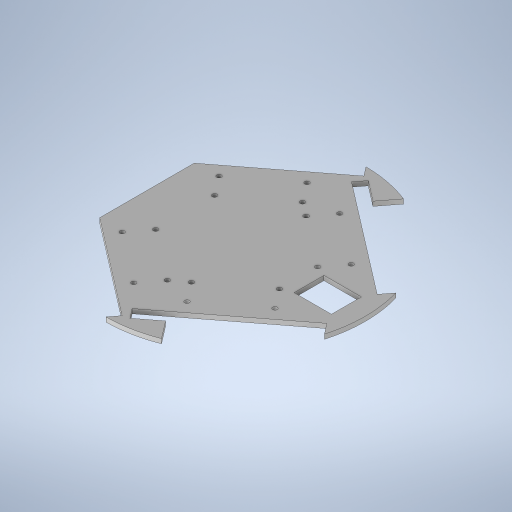
# Autodesk Inventor part: newbasecentral
Saved by Autodesk Inventor 2023.1 (Build 271208000, 208)
## iProperties
Created: 2022-09-07
Part Number: newbasecentral
Material: Genérico
Document SubType Name: Modeling
Designer: Lab. de Manufactura
Density: 1 g/cm^3
Appearance: Valor por defecto
Author: Lab. de Manufactura
Autodesk Inventor part; units mm, degrees
ref_plane "YZ Plane" through (0, 0, 0) normal (1, 0, 0) x (0, 1, 0)
ref_plane "XZ Plane" through (0, 0, 0) normal (0, 1, 0) x (-1, 0, 0)
ref_plane "XY Plane" through (0, 0, 0) normal (0, 0, 1) x (1, 0, 0)
sketch "Boceto1" plane through (0, 0, 0) normal (0, 1, 0) x (-1, 0, 0)
  line L0 (0, 0) -> (0, -87) construction
  line L1 (0, 0) -> (0, 83.8978) construction
  line L2 (0, 0) -> (-87, 0) construction
  line L3 (0, 0) -> (59, 0) construction
  line L4 (-74.5, -10) -> (-49.5, -10)
  line L5 (-49.5, -10) -> (-49.5, 10)
  line L6 (-49.5, 10) -> (-74.5, 10)
  line L7 (-74.5, 10) -> (-74.5, -10)
  line L8 (-74.5, -10) -> (-49.5, 10) construction
  line L9 (-49.5, -10) -> (-74.5, 10) construction
  line L10 (-18, 63.0769) -> (-64.0145, 27.7688)
  line L11 (9, 69.9829) -> (55.0145, 34.6747)
  line L12 (9, 69.9829) -> (20.2282, 84.6157)
  line L13 (-18, 63.0769) -> (-31.752, 80.9988)
  line L14 (-64.0145, 27.7688) -> (-75.6609, 42.9467)
  line L15 (-18, -63.0769) -> (-64.0145, -27.7688)
  line L16 (9, -69.9829) -> (55.0145, -34.6747)
  line L17 (9, -69.9829) -> (20.2282, -84.6157)
  line L18 (-18, -63.0769) -> (-31.752, -80.9988)
  line L19 (-64.0145, -27.7688) -> (-75.6609, -42.9467)
  arc A0 (-75.6609, 42.9467) -> (-75.6609, -42.9467) centre (0, 0) ccw
  arc A1 (20.2282, 84.6157) -> (-31.752, 80.9988) centre (0, 0) ccw
  arc A2 (-31.752, -80.9988) -> (20.2282, -84.6157) centre (0, 0) ccw
  line L20 (59, 37.9189) -> (59, -37.9189)
  line L21 (58.0583, 38.6415) -> (59, 37.9189)
  line L22 (55.0145, 34.6747) -> (58.0583, 38.6415)
  line L23 (58.0583, -38.6415) -> (59, -37.9189)
  line L24 (55.0145, -34.6747) -> (58.0583, -38.6415)
  circle A3 centre (-18.868, 51.0667) radius 1.5
  circle A4 centre (-52.1888, 25.4987) radius 1.5
  line L25 (-41.0072, 45.4229) -> (-35.5284, 38.2827) construction
  line L26 (-18.868, 51.0667) -> (-52.1888, 25.4987) construction
  line L27 (32.0072, 52.3288) -> (22.9685, 40.5493) construction
  circle A5 centre (9.868, 57.9726) radius 1.5
  circle A6 centre (43.1888, 32.4046) radius 1.5
  circle A7 centre (-18.868, -51.0667) radius 1.5
  circle A8 centre (-52.1888, -25.4987) radius 1.5
  circle A9 centre (9.868, -57.9726) radius 1.5
  circle A10 centre (43.1888, -32.4046) radius 1.5
  line L28 (43.1888, 32.4046) -> (9.868, 57.9726) construction
  point P0 (-62, 0)
  point P1 (-74.5, 0)
  point P2 (26.5284, 45.1886)
  dimension "d1" = 25
  dimension "d2" = 20
  dimension "d9" = 52.5
  dimension "d10" = 52.5
  dimension "d11" = 61
  dimension "d12" = 61
  dimension "d13" = 58
  dimension "d17" = 90
  dimension "d18" = 9
  dimension "d19" = 18
  dimension "d20" = 58
  dimension "d21" = 90
  dimension "d22" = 90
  dimension "d23" = 87
  dimension "d24" = 87
  dimension "d26" = 59
  dimension "d27" = 5
  dimension "d28" = 5
  dimension "d29" = 3
  dimension "d30" = 3
  dimension "d31" = 42
  dimension "d32" = 9
  dimension "d37" = 90
  dimension "d38" = 3
  dimension "d39" = 3
  dimension "d40" = 42
  dimension "d41" = 9
  dimension "d54" = 62
  constraints: 58 end point, 11 centre point, 11 symmetric about line, 9 parallel, 8 point on circle, 7 midpoint, 3 horizontal, 3 vertical, 2 perpendicular, 2 point on line, 1 coincident, 4 other
  measures "d1" distance of L5.end L6.end
  measures "d2" distance of L4.end L5.end
  measures "d9" angle of L1 L11
  measures "d10" angle of L1 L10
  measures "d11" distance from line of point (0, 0) L11
  measures "d12" distance from line of point (0, 0) L10
  measures "d13" distance of L11.start L11.end
  measures "d17" angle of L11 L12
  measures "d18" distance from line of L1 L11.start
  measures "d19" distance from line of L1 L10.start
  measures "d20" distance of L10.start L10.end
  measures "d21" angle of L10 L13
  measures "d22" angle of L10 L14
  measures "d23" radius of A0
  measures "d24" radius of A1
  measures "d26" distance between parallel lines of L0 L20
  measures "d27" distance between parallel lines of L11 L21
  measures "d28" distance between parallel lines of L23 L16
  measures "d29" diameter of A3
  measures "d30" diameter of A4
  measures "d31" distance of L26.end L26.start
  measures "d32" distance from line of L10 L26.start
  measures "d37" angle of L11 L27
  measures "d38" diameter of A5
  measures "d39" diameter of A6
  measures "d40" distance of L28.end L28.start
  measures "d41" distance from line of L11 L28.end
  measures "d54" distance of point (0, 0) point (-62, 0)
extrude "Extrusión1" add sketch "Boceto1" along normal blind 3
sketch "Boceto2" plane through (0, 3, 0) normal (0, 1, 0) x (1, 0, 0)
  line L0 (-55.0145, -34.6747) -> (-9, -69.9829) projected
  line L1 (-32.0072, -52.3288) -> (-0.1642, -10.8301) construction
  circle A0 centre (-33.4486, -19.711) radius 1.55
  circle A1 centre (-0.1278, -45.2789) radius 1.55
  line L2 (-33.4486, -19.711) -> (-0.1278, -45.2789) construction
  circle A2 centre (-43.1888, -32.4046) radius 1.5 construction
  line L3 (18, -63.0769) -> (64.0145, -27.7688) projected
  line L4 (41.0072, -45.4229) -> (14.3892, -10.7335) construction
  circle A3 centre (9.1278, -38.373) radius 1.55
  circle A4 centre (42.4486, -12.805) radius 1.55
  line L5 (42.4486, -12.805) -> (9.1278, -38.373) construction
  circle A5 centre (18.868, -51.0667) radius 1.5 construction
  line L6 (-59, 37.9189) -> (-59, -37.9189) construction
  line L7 (-59, 0) -> (115.874, 0) construction
  circle A6 centre (-33.4486, 19.711) radius 1.55
  circle A7 centre (-0.1278, 45.2789) radius 1.55
  circle A8 centre (9.1278, 38.373) radius 1.55
  circle A9 centre (42.4486, 12.805) radius 1.55
  point P0 (0, 0)
  dimension "d44" = 3.1
  dimension "d45" = 3.1
  dimension "d46" = 21
  dimension "d47" = 42
  dimension "d48" = 16
  dimension "d51" = 16
  dimension "d52" = 21
  dimension "d53" = 42
  constraints: 10 end point, 8 centre point, 4 symmetric about line, 3 midpoint, 2 equal radius, 2 parallel, 2 perpendicular, 1 horizontal, 4 other
  measures "d44" diameter of A0
  measures "d45" diameter of A1
  measures "d46" distance from line of L1 L2.start
  measures "d47" distance of L2.start L2.end
  measures "d48" distance of A2.centre L2.start
  measures "d51" distance from line of L5 A5.centre
  measures "d52" distance from line of L4 L5.end
  measures "d53" distance of L5.start L5.end
extrude "Extrusión2" cut sketch "Boceto2" against normal blind 10
sketch "Boceto3" plane through (0, 3, 0) normal (0, 1, 0) x (1, 0, 0)
  circle A0 centre (0, 0) radius 90 construction
  dimension "d55" = 180
  constraints: 1 centre point, 1 coincident
  measures "d55" diameter of A0
sketch "Boceto5" plane through (0, 3, 0) normal (0, 1, 0) x (1, 0, 0)
  arc A0 (75.6609, -42.9467) -> (75.6609, 42.9467) centre (0, 0) ccw construction
  line L0 (87, 0) -> (-107.1861, 0) construction
  line L1 (-55.0145, -34.6747) -> (-9, -69.9829) projected
  line L2 (-9, -69.9829) -> (5.2804, -80.9406)
  line L3 (5.2804, -80.9406) -> (0.6326, -86.9977)
  arc A1 (-20.2282, -84.6157) -> (31.752, -80.9988) centre (0, 0) ccw projected
  line L4 (31.752, -80.9988) -> (18, -63.0769) projected
  line L5 (18, -63.0769) -> (4.513, -73.4259)
  line L6 (4.513, -73.4259) -> (9.3831, -79.7727)
  line L7 (9.3831, -79.7727) -> (22.8701, -69.4238)
  line L8 (-55.0145, -34.6747) -> (-59, -31.6165)
  line L9 (-59, 37.9189) -> (-59, -37.9189) projected
  circle A2 centre (42.4486, 12.805) radius 1.55 projected
  circle A3 centre (-33.4486, -19.711) radius 1.55 projected
  circle A4 centre (-33.4486, 19.711) radius 1.55 projected
  circle A5 centre (42.4486, -12.805) radius 1.55 projected
  circle A6 centre (9.1278, 38.373) radius 1.55 projected
  circle A7 centre (-0.1278, -45.2789) radius 1.55 projected
  circle A8 centre (-0.1278, 45.2789) radius 1.55 projected
  circle A9 centre (9.1278, -38.373) radius 1.55 projected
  arc A10 (-20.2282, -84.6157) -> (31.752, -80.9988) centre (0, 0) ccw projected
  line L10 (31.752, -80.9988) -> (18, -63.0769) projected
  line L11 (18, -63.0769) -> (64.0145, -27.7688) projected
  line L12 (64.0145, -27.7688) -> (75.6609, -42.9467) projected
  arc A11 (75.6609, -42.9467) -> (75.6609, 42.9467) centre (0, 0) ccw projected
  line L13 (75.6609, 42.9467) -> (64.0145, 27.7688) projected
  line L14 (64.0145, 27.7688) -> (18, 63.0769) projected
  line L15 (18, 63.0769) -> (31.752, 80.9988) projected
  arc A12 (31.752, 80.9988) -> (-20.2282, 84.6157) centre (0, 0) ccw projected
  line L16 (-20.2282, 84.6157) -> (-9, 69.9829) projected
  line L17 (-9, 69.9829) -> (-55.0145, 34.6747) projected
  line L18 (-55.0145, 34.6747) -> (-58.0583, 38.6415) projected
  line L19 (-58.0583, 38.6415) -> (-59, 37.9189) projected
  line L20 (-59, 37.9189) -> (-59, -37.9189) projected
  line L21 (-59, -37.9189) -> (-58.0583, -38.6415) projected
  line L22 (-58.0583, -38.6415) -> (-55.0145, -34.6747) projected
  line L23 (-55.0145, -34.6747) -> (-9, -69.9829) projected
  line L24 (-9, -69.9829) -> (-20.2282, -84.6157) projected
  circle A13 centre (-43.1888, 32.4046) radius 1.5 projected
  circle A14 centre (-9.868, 57.9726) radius 1.5 projected
  circle A15 centre (18.868, 51.0667) radius 1.5 projected
  circle A16 centre (52.1888, 25.4987) radius 1.5 projected
  circle A17 centre (-43.1888, -32.4046) radius 1.5 projected
  circle A18 centre (-9.868, -57.9726) radius 1.5 projected
  circle A19 centre (52.1888, -25.4987) radius 1.5 projected
  circle A20 centre (18.868, -51.0667) radius 1.5 projected
  line L25 (74.5, 10) -> (74.5, -10) projected
  line L26 (74.5, -10) -> (49.5, -10) projected
  line L27 (49.5, -10) -> (49.5, 10) projected
  line L28 (49.5, 10) -> (74.5, 10) projected
  line L29 (18, -63.0769) -> (64.0145, -27.7688) projected
  line L30 (64.0145, -27.7688) -> (78.2949, -16.8111)
  line L31 (78.2949, -16.8111) -> (83.6749, -23.8225)
  point P0 (-9, -69.9829)
  point P1 (-20.2282, -84.6157)
  dimension "d66" = 18
  dimension "d67" = 17
  dimension "d68" = 8
  dimension "d69" = 18
  constraints: 18 end point, 5 perpendicular, 3 collinear, 3 point on circle, 2 point on line, 1 horizontal
  measures "d66" distance of L1.end L2.end
  measures "d67" distance of L4.end L5.end
  measures "d68" distance of L5.end L6.end
  measures "d69" distance of L11.end L30.end
extrude "Extrusión3" cut sketch "Boceto5" against normal blind 10 contours L22 L21 L9 L8 | L2 L3 A1 L24 | L7 L6 L5 L4 | L30 L31 A11 L12
mirror "Simetría1" about plane through (0, 0, 0) normal (0, 0, 1) of "Extrusión3"
ref_plane "Plano de trabajo1" through (0, 0, 0) normal (0, 0, 1) x (1, 0, 0)
